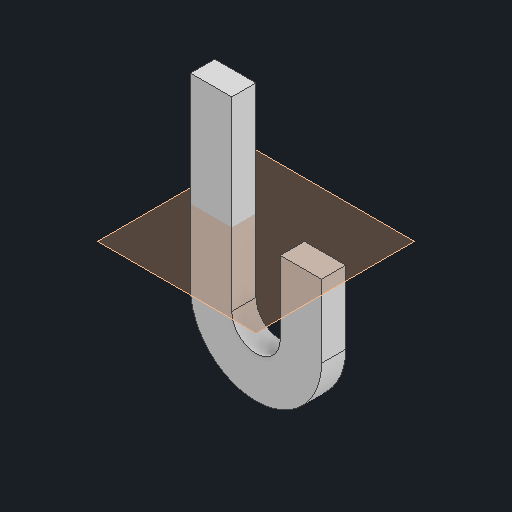
# Autodesk Inventor part: joint
Saved by Autodesk Inventor 2022 (Build 260153000, 153)
## iProperties
Created: 2023-02-06
Part Number: joint
Material: Generic
Document SubType Name: Modeling
Designer: erwin
Density: 1 g/cm^3
Appearance: Default
Author: erwin
Autodesk Inventor part; units mm, degrees
ref_plane "YZ Plane" through (0, 0, 0) normal (1, 0, 0) x (0, 1, 0)
ref_plane "XY Plane" through (0, 0, 0) normal (0, 0, 1) x (1, 0, 0)
sketch "Sketch1" plane through (0, 0, 0) normal (0, 0, 1) x (1, 0, 0)
  line L0 (0.75, 11.8) -> (0.75, -11.8) projected
  arc A0 (0.75, 11.8) -> (-0.95, 11.8) centre (-0.1, 11.8) ccw projected
  line L1 (-0.95, -11.8) -> (-0.95, 11.8) projected
  arc A1 (-0.95, -11.8) -> (0.75, -11.8) centre (-0.1, -11.8) ccw projected
  line L2 (-2.95, 12.1582) -> (-2.95, -7.1418) projected
  arc A2 (-2.95, 12.1582) -> (-4.65, 12.1582) centre (-3.8, 12.1582) ccw projected
  line L3 (-4.65, -7.1418) -> (-4.65, 12.1582) projected
  arc A3 (-4.65, -7.1418) -> (-2.95, -7.1418) centre (-3.8, -7.1418) ccw projected
  line L4 (-3.8, -7.1418) -> (-3.8, -10.1418)
  line L5 (-0.1, -14.8) -> (-0.1, -11.8)
  arc A4 (-3.8, -14.8004) -> (-0.1, -14.8) centre (-1.95, -14.8) ccw
  line L6 (-3.8, -14.8004) -> (-3.8, -10.1418)
  point P0 (0, 0)
  dimension "d0" = 3
  dimension "d1" = 3
  constraints: 6 end point, 2 point on circle, 1 centre point, 1 collinear, 1 parallel, 1 tangent, 1 vertical
  measures "d0" distance of L5.start L5.end
  measures "d1" distance of L4.start L4.end
ref_plane "Work Plane1" through (-0.1, -11.8, 0) normal (0, 1, 0) x (-1, 0, 0)
sketch "Sketch2" plane through (-0.1, -11.8, 0) normal (0, 1, 0) x (-1, 0, 0)
  line L0 (0.85, -1) -> (-0.85, -1)
  line L1 (-0.85, -1) -> (-0.85, 0)
  line L2 (-0.85, 0) -> (0.85, 0)
  line L3 (0.85, 0) -> (0.85, -1)
  line L4 (-0.85, 0) -> (0.85, 0) projected
  point P0 (-0.1, 0)
  point P1 (0, 0)
  dimension "d2" = 1.7
  dimension "d3" = 1
  constraints: 8 end point, 2 midpoint, 2 parallel, 1 horizontal, 1 perpendicular
  measures "d2" distance of L0.start L0.end
  measures "d3" distance of L2.end L0.start
sweep "Sweep1" add profiles "Sketch2" path "Sketch1" path curves L5 A4 L6 L4
equation "\"d1\" = d0"
body "Solid1"
